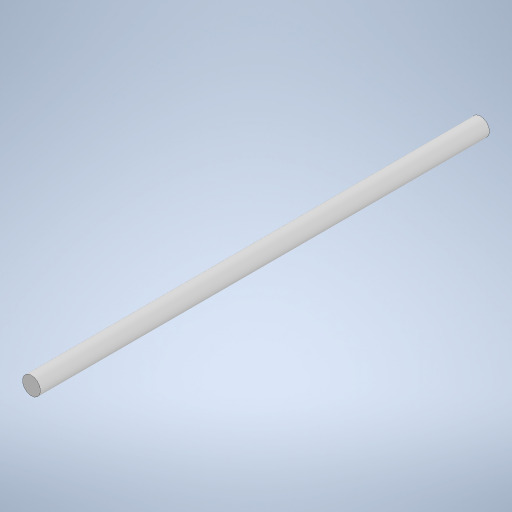
# Autodesk Inventor part: Bauteile 1
Saved by Autodesk Inventor 2023 (Build 270158000, 158)
## iProperties
Created: 2024-02-02
Part Number: Bauteile 1
Material: Generisch
Document SubType Name: Modeling
Designer: jefar
Density: 1 g/cm^3
Appearance: Vorgabe
Author: jefar
Autodesk Inventor part; units mm, degrees
ref_plane "YZ Plane" through (0, 0, 0) normal (1, 0, 0) x (0, 1, 0)
ref_plane "XZ Plane" through (0, 0, 0) normal (0, 1, 0) x (-1, 0, 0)
ref_plane "XY Plane" through (0, 0, 0) normal (0, 0, 1) x (1, 0, 0)
sketch "Skizze1" plane through (0, 0, 0) normal (0, 0, 1) x (1, 0, 0)
  line L0 (-280, 0) -> (280, 0) construction
  line L1 (0, -280) -> (0, 280) construction
  circle A0 centre (0, 0) radius 200
  dimension "d2" = 400
  constraints: 1 centre point, 1 coincident
  measures "d2" diameter of A0
sketch "Skizze2" plane through (0, 0, 0) normal (1, 0, 0) x (0, 1, 0)
  point P0 (0, 0)
extrude "Extrusion1" add sketch "Skizze1" along normal blind 10000
